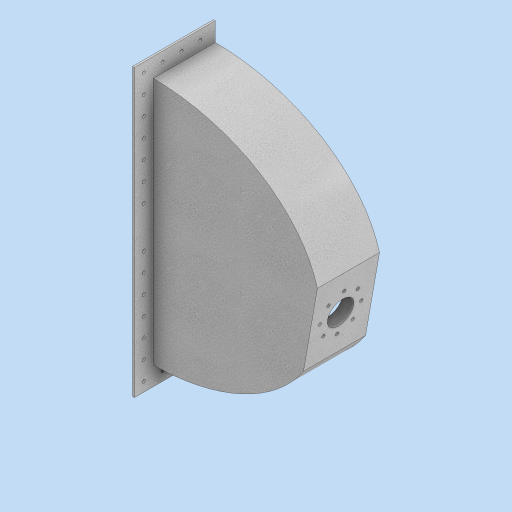
# Autodesk Inventor part: eggshellCorePrinted
Saved by Autodesk Inventor 2023 (Build 270158000, 158)
## iProperties
Created: 2026-03-19
Part Number: eggshellCorePrinted
Material: GFRC
Document SubType Name: Modeling
Designer: Nathann
Density: 1.7 g/cm^3
Appearance: Flat - Polished Gray
Mass: 6774.09 g
Surface Area: 8560.51 cm^2
Volume: 6774.09 cm^3
Author: Nathann
Autodesk Inventor part; units mm, degrees
ref_plane "YZ Plane" through (0, 0, 0) normal (1, 0, 0) x (0, 1, 0)
ref_plane "XZ Plane" through (0, 0, 0) normal (0, 1, 0) x (-1, 0, 0)
ref_plane "XY Plane" through (0, 0, 0) normal (0, 0, 1) x (1, 0, 0)
sketch "Sketch1" plane through (0, 0, 0) normal (0, 0, 1) x (1, 0, 0)
  ellipse E0 centre (0, 0) end of major axis (0, 330) minor radius 450 (0, -330) -> (0, 330) ccw
  ellipse E1 centre (0, 0) end of major axis (420, 0) minor radius 300 (0, -300) -> (0, 300) ccw
  line L0 (0, 300) -> (0, 330)
  line L1 (0, -300) -> (0, -330)
  line L2 (420, 0) -> (450, 0)
  dimension "d0" = 420
  dimension "d1" = 450
  dimension "d2" = 300
  dimension "d3" = 330
  constraints: 6 end point, 2 coincident, 2 point on line, 1 horizontal, 10 other
extrude "Extrusion1" add sketch "Sketch1" along normal blind 160
sketch "Sketch3" plane through (0, 0, 0) normal (0, 0, -1) x (-1, 0, 0)
  ellipse E0 centre (0, 0) end of major axis (420, 0) minor radius 300 (0, 300) -> (0, -300) ccw projected
  line L0 (-410.6033, 63.104) -> (-375.8737, -133.8576)
  line L1 (-375.8737, -133.8576) -> (-428.5073, -143.1383)
  line L2 (-428.5073, -143.1383) -> (-456.291, 14.4309)
  line L3 (0, 300) -> (0, -300) projected
  ellipse E1 centre (0, 0) end of major axis (450, 0) minor radius 330 (0, 330) -> (0, -330) ccw projected
  line L4 (-456.291, 14.4309) -> (-439.6592, 70.3382)
  line L5 (-428.5073, -143.1383) -> (-336.4493, -219.1451)
  line L6 (-336.4493, -219.1451) -> (-375.8737, -133.8576)
  line L7 (-410.6033, 63.104) -> (-439.6592, 70.3382)
  line L8 (-393.2385, -35.3768) -> (260.9914, 90.2506)
  line L9 (260.9914, 90.2506) -> (260.9914, 44.7879)
  line L10 (260.9914, 44.7879) -> (0, 40.1342)
  dimension "d8" = 200
  dimension "d9" = 10
  dimension "d12" = 45.4627
  dimension "d13" = 160
  constraints: 20 end point, 2 perpendicular, 2 point on line, 1 midpoint, 1 vertical, 9 other
  measures "d8" distance of L0.start L0.end
  measures "d9" angle of L3 L0
  measures "d12" distance of L8.end L9.end
  measures "d13" distance of L1.end L2.end
extrude "Extrusion2" add sketch "Sketch3" against normal blind 160 contours L0 E0
sketch "Sketch7" plane through (0, 0, 160) normal (0, 0, 1) x (1, 0, 0)
  ellipse E0 centre (0, 0) end of major axis (-450, 0) minor radius 330 (0, -330) -> (0, 330) ccw projected
  line L0 (0, 330) -> (0, 300) projected
  ellipse E1 centre (0, 0) end of major axis (-420, 0) minor radius 300 (410.6033, 63.104) -> (0, 300) ccw projected
  line L1 (410.6033, 63.104) -> (375.8737, -133.8576) projected
  ellipse E2 centre (0, 0) end of major axis (-420, 0) minor radius 300 (0, -300) -> (375.8737, -133.8576) ccw projected
  line L2 (0, -300) -> (0, -330) projected
  line L3 (0, -300) -> (0, 300)
  constraints: 2 end point, 1 vertical, 3 other
extrude "Extrusion6" add sketch "Sketch7" along normal blind 5
ref_plane "Work Plane2" through (405.4179, -139.067, 0) normal (-0.9848078, 0.1736482, 0) x (0, 0, 1)
sketch "Sketch8" plane through (405.4179, -139.067, 0) normal (-0.9848078, 0.1736482, 0) x (0, 0, 1)
  circle A0 centre (80.8275, 83.1092) radius 366.3368
  point P0 (0, 66.5542)
  constraints: 1 centre point
extrude "Extrusion7" cut sketch "Sketch8" against normal blind 200
sketch "Sketch9" plane through (0, 300, 0) normal (-1, 0, 0) x (0, 0, 1)
  line L0 (0, -630) -> (0, -444.7158) projected
  line L1 (0, -630) -> (215, -630)
  line L2 (215, -630) -> (215, -680)
  line L3 (215, -680) -> (0, -680)
  line L4 (0, -680) -> (0, -630)
  line L5 (165, -235.481) -> (165, 30) projected
  line L6 (215, -630) -> (165, -630)
  line L7 (165, -630) -> (165, 30)
  line L8 (165, 30) -> (215, 30)
  line L9 (215, 30) -> (215, -630)
  line L10 (215, 30) -> (0, 30)
  line L11 (0, 30) -> (0, 80)
  line L12 (0, 80) -> (215, 80)
  line L13 (215, 80) -> (215, 30)
  circle A0 centre (190, -655) radius 4.5
  circle A1 centre (140, -655) radius 4.5
  circle A2 centre (90, -655) radius 4.5
  circle A3 centre (40, -655) radius 4.5
  circle A4 centre (190, -605) radius 4.5
  circle A5 centre (190, -555) radius 4.5
  circle A6 centre (190, -505) radius 4.5
  circle A7 centre (190, -455) radius 4.5
  circle A8 centre (190, -405) radius 4.5
  circle A9 centre (190, -355) radius 4.5
  line L14 (215, -300) -> (251.9501, -300)
  circle A10 centre (190, 55) radius 4.5
  circle A11 centre (140, 55) radius 4.5
  circle A12 centre (90, 55) radius 4.5
  circle A13 centre (40, 55) radius 4.5
  circle A14 centre (190, 5) radius 4.5
  circle A15 centre (190, -45) radius 4.5
  circle A16 centre (190, -95) radius 4.5
  circle A17 centre (190, -145) radius 4.5
  circle A18 centre (190, -195) radius 4.5
  circle A19 centre (190, -245) radius 4.5
  point P0 (0, -300)
  dimension "d34" = 50
  dimension "d35" = 50
  dimension "d36" = 50
  dimension "d39" = 9
  dimension "d40" = 25
  dimension "d41" = 25
  dimension "d44" = 50
  dimension "d51" = 50
  constraints: 26 end point, 20 centre point, 10 symmetric about line, 6 parallel, 5 horizontal, 3 perpendicular, 1 midpoint, 1 point on line, 1 vertical, 28 other
  measures "d34" distance between parallel lines of L7 L9
  measures "d35" distance between parallel lines of L3 L1
  measures "d36" distance between parallel lines of L8 L12
  measures "d39" diameter of A0
  measures "d40" distance from line of L3 A0.centre
  measures "d41" distance from line of L2 A0.centre
  measures "d44" distance of A0.centre A1.centre
  measures "d51" distance of A0.centre A4.centre
sketch "Sketch10" plane through (0, 300, 0) normal (-1, 0, 0) x (0, 0, 1)
  point P0 (0, -300)
extrude "Extrusion8" add sketch "Sketch9" against normal blind 5
sketch "Sketch11" plane through (405.4179, -139.067, 0) normal (0.9848078, -0.1736482, 0) x (0, 0, -1)
  circle A0 centre (-85, 100.4954) radius 35
  circle A1 centre (-85, 155.4954) radius 4.5
  line L0 (0, -5.7359) -> (-165, -5.7359) projected
  line L1 (-165, 206.7266) -> (0, 206.7266) projected
  line L2 (-165, -5.7359) -> (-165, 206.7266) projected
  circle A2 centre (-123.8909, 139.3862) radius 4.5
  circle A3 centre (-140, 100.4954) radius 4.5
  circle A4 centre (-123.8909, 61.6045) radius 4.5
  circle A5 centre (-85, 45.4954) radius 4.5
  circle A6 centre (-46.1091, 61.6045) radius 4.5
  circle A7 centre (-30, 100.4954) radius 4.5
  circle A8 centre (-46.1091, 139.3862) radius 4.5
  point P0 (0, 66.5542)
  dimension "d56" = 70
  dimension "d57" = 9
  dimension "d58" = 55
  dimension "d59" = 212.4625
  dimension "d60" = 106.2313
  dimension "d61" = 80
  dimension "d64" = 360
  dimension "d66" = 0
  constraints: 9 centre point, 17 other
  measures "d56" diameter of A0
  measures "d57" diameter of A1
  measures "d58" distance of A0.centre A1.centre
  measures "d59" distance between parallel lines of L0 L1
  measures "d60" distance from line of L1 A0.centre
  measures "d61" distance from line of L2 A0.centre
  measures "d66" horizontal distance of A1.centre A0.centre
extrude "Extrusion9" cut sketch "Sketch11" against normal blind 50
equation "\"d60\" = 0.5 * d59"
body "Solid1"
